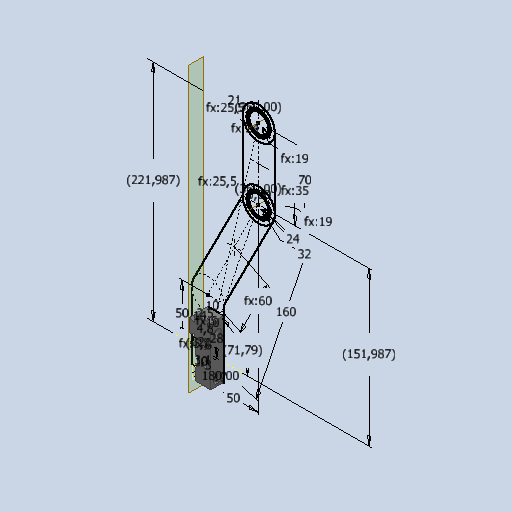
# Autodesk Inventor part: ParallelSystem_ProximalPart_Driven_Counterpart
Saved by Autodesk Inventor 2024 (Build 280153000, 153)
## iProperties
Created: 2022-07-18
Part Number: ParallelSystem_ProximalPart_Driven_Counterpart
Material: PBT-Kunststoff
Document SubType Name: Modeling
Designer: alexw
Density: 1.31 g/cm^3
Appearance: Glatt - Weiß
Mass: 124.576 g
Surface Area: 279.297 cm^2
Volume: 95.0965 cm^3
d4: 25,000 mm
d7: 5,000 mm
d9: 6,000 mm
d10: 0,00 grd
d11: 25,000 mm
d23: 8,000 mm
d36: 0,00 grd
d37: 30,000 mm
d40: 120,000 mm
d41: 50,000 mm
d42: 60,000 mm
d43: 19,000 mm
d44: 12,000 mm
d45: 35,000 mm
Passfeder_width: 3,000 mm
Nabennuttiefe: 1,400 mm
ParallelLink_BearingStep_Height: 10,000 mm
ParallelLink_Lever_Thickness: 8,000 mm
ParallelHebel_Gabelgelenk_OuterDia: 32,000 mm
Nadellager_OuterDia: 19,000 mm
ParallelHebel_Passflansch_HoleDia: 25,500 mm
d65: 3,000 oE
d69: 25,500 mm
d70: 3,000 oE
Distanze_daVinciHead_Pivot: 221,987 mm
Lager_Einbautiefe: 5,000 mm
Lager_Bohrung_Durchmesser: 19,000 mm
Support_Link_Length: 160,000 mm
ParallelMech_LINK_GabelDist: 70,000 mm
VerticalDistance: 70,000 mm
Author: alexw
Autodesk Inventor part; units mm, degrees
note: some values were not read from the file. Chosen so that the rebuilt part matches the saved one: direction of "Bohrung6".
ref_plane "YZ Plane" through (0, 0, 0) normal (1, 0, 0) x (0, 1, 0)
ref_plane "XZ Plane" through (0, 0, 0) normal (0, 1, 0) x (-1, 0, 0)
sketch "Skizze1" plane through (0, 0, 0) normal (0, 0, 1) x (1, 0, 0)
  line L0 (-33.0017, 0) -> (83.0017, 0) construction
  circle A0 centre (50, 151.9868) radius 16
  line L1 (66, 151.9868) -> (66, 221.9868)
  line L2 (34, 151.9868) -> (34, 221.9868)
  line L3 (50, 151.9868) -> (50, 237.9868) construction
  line L4 (50, 151.9868) -> (50, 167.9868) construction
  line L5 (34, 151.9868) -> (66, 151.9868) construction
  line L6 (-16, 0) -> (-16, 50)
  line L7 (16, 0) -> (16, 50)
  line L8 (-16, 50) -> (16, 50) construction
  circle A1 centre (0, 50) radius 16 construction
  line L9 (-14.2566, 57.2629) -> (34, 151.9868)
  arc A2 (-14.2566, 57.2629) -> (-16, 50) centre (0, 50) ccw
  line L10 (16, 50) -> (64.2566, 144.7239)
  arc A3 (64.2566, 144.7239) -> (66, 151.9868) centre (50, 151.9868) ccw
  line L11 (0, 50) -> (50, 151.9868) construction
  circle A4 centre (50, 221.9868) radius 16
  circle A5 centre (50, 221.9868) radius 9.5
  circle A6 centre (50, 151.9868) radius 9.5
  line L12 (0, 0) -> (0, 5) construction
  circle A7 centre (50, 151.9868) radius 12.75 construction
  circle A8 centre (50, 221.9868) radius 12.75 construction
  line L13 (0, 0) -> (50, 221.9868) construction
  circle A9 centre (50, 221.9868) radius 10.5
  circle A10 centre (50, 151.9868) radius 10.5
  circle A11 centre (50, 151.9868) radius 12
  circle A12 centre (50, 221.9868) radius 12
  line L14 (-16, 0) -> (-16, -17)
  line L15 (-16, -17) -> (16, -17)
  line L16 (16, -17) -> (16, 0)
  circle A13 centre (0, 0) radius 5
  line L17 (-1.5, -4.7697) -> (-1.5, -17)
  line L18 (1.5, -17) -> (1.5, -4.7697)
  line L19 (-16, 0) -> (16, 0) construction
  arc A14 (16, 0) -> (-16, 0) centre (0, 0) ccw
  line L20 (-1.5, 4.7697) -> (-1.5, 10.7697)
  arc A15 (1.5, 10.7697) -> (-1.5, 10.7697) centre (0, 10.7697) ccw
  line L21 (1.5, 10.7697) -> (1.5, 4.7697)
  line L22 (1.5, 4.7697) -> (-1.5, 4.7697)
  line L23 (0, 12.2697) -> (0, 40)
  line L24 (0, 40) -> (16, 40)
  line L25 (0, 33) -> (-4.8, 35)
  line L26 (-4.8, 35) -> (-4.8, 21)
  line L27 (-4.8, 21) -> (0, 23)
  line L28 (-4.8, 28) -> (0, 28) construction
  line L29 (-4.8, 30.5) -> (0, 30.5) construction
  line L30 (-4.8, 25.5) -> (0, 25.5) construction
  circle A16 centre (-10.5, 0) radius 1.55
  circle A17 centre (10.5, 0) radius 1.55
  line L31 (0, 0) -> (50, 151.9868) construction
  point P0 (26.4122, 103.8739)
  point P1 (50, 186.9868)
  point P2 (50, 164.7368)
  point P3 (38.9582, 145.6118)
  point P4 (61.0418, 145.6118)
  point P5 (50, 234.7368)
  point P6 (38.9582, 215.6118)
  point P7 (61.0418, 215.6118)
  point P8 (-5, 0)
  dimension "d69" = 25.5
  dimension "ParallelHebel_Passflansch_HoleDia" = 25.5
  dimension "d36" = 0
  dimension "ParallelHebel_Gabelgelenk_OuterDia" = 32
  dimension "VerticalDistance" = 70
  dimension "d42" = 60
  dimension "d43" = 19
  dimension "Nadellager_OuterDia" = 19
  dimension "d45" = 35
  dimension "d67" = 360
  dimension "d72" = 360
  dimension "Distanze_daVinciHead_Pivot" = 221.9868
  dimension "d88" = 21
  dimension "d91" = 24
  dimension "d92" = 24
  dimension "d97" = 151.9868
  dimension "Support_Link_Length" = 160
  dimension "d100" = 10
  dimension "d101" = 3
  dimension "d102" = 0
  dimension "d103" = 17
  dimension "d105" = 32
  dimension "d125" = 50
  dimension "d128" = 50
  dimension "d138" = 6
  dimension "d139" = 10
  dimension "d142" = 14
  dimension "d143" = 10
  dimension "d144" = 2.5
  dimension "d145" = 5
  dimension "d146" = 4.8
  dimension "d147" = 28
  dimension "d173" = 11
  dimension "d174" = 5.5
  dimension "d175" = 3.1
  dimension "d178" = 71.79
  constraints: 62 end point, 26 point on circle, 22 point on line, 16 centre point, 16 tangent, 12 coincident, 9 perpendicular, 5 vertical, 4 midpoint, 3 equal length, 3 equal radius, 3 horizontal, 3 parallel, 2 collinear, 2 symmetric about line, 2 vertical alignment, 13 other
  measures "d36" distance between parallel lines of L3 L4
  measures "ParallelHebel_Gabelgelenk_OuterDia" diameter of A0
  measures "VerticalDistance" distance of A4.centre point (50, 151.987)
  measures "d42" distance of point (26.412, 103.874) A1.centre
  measures "d43" diameter of A5
  measures "Nadellager_OuterDia" diameter of A6
  measures "d45" distance of point (50, 186.987) point (50, 151.987)
  measures "Distanze_daVinciHead_Pivot" distance from line of A4.centre L0
  measures "d88" diameter of A9
  measures "d91" diameter of A11
  measures "d92" diameter of A12
  measures "d97" vertical distance of point (50, 151.987) L12.start
  measures "Support_Link_Length" distance of A0.centre L12.start
  measures "d100" diameter of A13
  measures "d101" distance between parallel lines of L18 L17
  measures "d102" angle of L16 L14
  measures "d103" distance between parallel lines of L15 L19
  measures "d105" diameter of A14
  measures "d125" distance of L12.start L11.start
  measures "d128" horizontal distance of L12.start point (50, 151.987)
  measures "d138" distance from line of L22 A15.centre
  measures "d139" distance between parallel lines of L8 L24
  measures "d142" distance of L25.end L26.end
  measures "d143" distance of L27.end L25.start
  measures "d144" distance between parallel lines of L29 L28
  measures "d145" distance between parallel lines of L29 L30
  measures "d146" distance between parallel lines of L23 L26
  measures "d147" distance from line of L12.start L28
  measures "d173" distance of L6.start point (-5, 0)
  measures "d174" distance from line of L14 point (-10.5, 0)
  measures "d175" diameter of A16
  measures "d178" angle of L0 L31
extrude "Extrusion2" add sketch "Skizze1" along normal blind 8 contours A0 | A0 L2 A4 L1 | A0 L10 L7 L24 L23 L25 L26 L27 A14 L6 A2 L9 | A4 | L7 A14 L23 L24 | A14 L23 A15 L20 A13 L17 L15 L14 | L16 L15 L18 A13 L21 A15 L23 A14 | L23 L27 L26 L25 | A15 L21 A13 L20 | A9 | A10 | A11 | A12 | A16 | A17
fillet "Rundung1" radius 25 2 edges at (34, 151.9868, 4) (16, 50, 4)
hole "Bohrung2" at (50, 186.9868, 0) at (26.4122, 103.8739, 0) direction (0, 0, 1) diameter 8 end through all
ref_plane "Arbeitsebene1" through (50, 151.9868, 0) normal (-1, 0, 0) x (0, 0, 1)
extrude "Extrusion6" cut sketch "Skizze1" along normal blind 1 contours A5 | A9 | A10 | A11 | A12
extrude "Extrusion7" cut sketch "Skizze1" along normal blind 1 from surface at 1 contours A9 | A10
sketch "Skizze8" plane through (0, 0, 8) normal (0, 0, 1) x (1, 0, 0)
  circle A0 centre (50, 186.9868) radius 4 projected
  circle A1 centre (26.4122, 103.8739) radius 4 projected
  arc A2 (64.2566, 144.7239) -> (66, 151.9868) centre (50, 151.9868) ccw projected
  line L0 (66, 151.9868) -> (66, 221.9868) projected
  arc A3 (66, 221.9868) -> (34, 221.9868) centre (50, 221.9868) ccw projected
  line L1 (34, 221.9868) -> (34, 157.988) projected
  arc A4 (31.2759, 146.6396) -> (34, 157.988) centre (9, 157.988) ccw projected
  line L2 (31.2759, 146.6396) -> (-14.2566, 57.2629) projected
  arc A5 (-14.2566, 57.2629) -> (-16, 50) centre (0, 50) ccw projected
  line L3 (-16, 50) -> (-16, -17) projected
  line L4 (-16, -17) -> (-1.5, -17) projected
  line L5 (-1.5, -17) -> (-1.5, -4.7697) projected
  arc A6 (1.5, -4.7697) -> (-1.5, -4.7697) centre (0, 0) ccw projected
  line L6 (1.5, -4.7697) -> (1.5, -17) projected
  line L7 (1.5, -17) -> (16, -17) projected
  line L8 (16, -17) -> (16, 43.9989) projected
  arc A7 (18.7241, 55.3472) -> (16, 43.9989) centre (41, 43.9989) ccw projected
  line L9 (18.7241, 55.3472) -> (64.2566, 144.7239) projected
  circle A8 centre (50, 151.9868) radius 9.5 projected
  circle A9 centre (50, 221.9868) radius 9.5 projected
extrude "Extrusion9" add sketch "Skizze8" along normal blind 5
sketch "Skizze5" plane through (-1.5, -17, 0) normal (1, 0, 0) x (0, 0, -1)
  line L0 (0, 0) -> (0, 12.2303) construction
  line L1 (0, 12.2303) -> (-13, 12.2303) construction
  line L2 (0, 0) -> (-13, 0) construction
  line L3 (-13, 12.2303) -> (0, 0) construction
  line L4 (-13, 0) -> (0, 12.2303) construction
  line L5 (-13, 0) -> (-13, 12.2303) construction
  point P0 (0, 17)
  point P1 (-6.5, 6.1152)
  constraints: 4 end point, 1 midpoint
extrude "Extrusion11" add sketch "Skizze1" along normal up to surface (13 mm away) separate body contours L7 A14 L23 L24 | L16 L15 L18 A13 L21 A15 L23 A14 | L23 L27 L26 L25 | A17
extrude "Extrusion10" cut sketch "Skizze1" along normal up to surface (13 mm away) contours L7 A14 L23 L24 | L16 L15 L18 A13 L21 A15 L23 A14 | L23 L27 L26 L25 | A15 L21 A13 L20 | A17 bodies 1
hole "Bohrung4" at (-1.5, -10.8848, 6.5) direction (-1, 0, 0) diameter 3.242 end through all bodies 1 thread size "M4x0.7" class "6H" standard "ISO Metric profile"
sketch "Skizze9" plane through (16, -17, 0) normal (1, 0, 0) x (0, 0, -1)
  point P0 (0, 17)
  point P1 (-6.5, 6.1152)
hole "Bohrung6" at (16, -10.8848, 6.5) direction (-1, 0, 0) diameter 4.5 depth 17.5 counterbore diameter 8 counterbore depth 4.5 bodies 2 clearance for "Inbusschraube DIN EN ISO 4762" size "M4" standard "DIN"
ref_plane "Arbeitsebene2" through (-4.8, 72.7467, 13) normal (-1, 0, 0) x (0, 1, 0)
sketch "Skizze12" plane through (-4.8, 72.7467, 13) normal (-1, 0, 0) x (0, 1, 0)
  line L0 (-44.7467, 13) -> (-44.7467, 6.5) construction
  line L1 (-22.7467, 13) -> (-89.7467, 13) construction
  line L2 (-22.7467, 0) -> (-89.7467, 0) construction
  point P0 (-72.7467, 13)
  point P1 (-44.7467, 13)
  dimension "d150" = 13
  dimension "d151" = 6.5
  constraints: 2 end point, 1 coincident, 1 vertical
  measures "d150" distance between parallel lines of L1 L2
  measures "d151" distance of L0.start L0.end
sketch "Skizze13" plane through (16, -17, 0) normal (1, 0, 0) x (0, 0, -1)
  point P0 (0, 17)
  point P1 (-6.5, 45)
hole "Bohrung7" at (-4.8, 28, 6.5) direction (-1, 0, 0) diameter 3.242 end through all bodies 1 thread size "M4x0.7" class "6H" standard "ISO Metric profile"
hole "Bohrung8" at (16, 28, 6.5) direction (-1, 0, 0) diameter 4.5 end through all counterbore diameter 8 counterbore depth 4.5 bodies 2 clearance for "Inbusschraube DIN EN ISO 4762" size "M4" standard "DIN"
extrude "Extrusion12" cut sketch "Skizze1" along normal through all contours A17 bodies 2
delete faces "Fläche löschen1" heal no whole lump yes faces at (-8.5333, 28.26, 4.9)
thicken "Thicken1" operation add thickness 0.15 both sides no extend neighbours yes toward (-0.3846154, -0.9230769, 0) bodies 2 faces at (-1.6, 33.6667, 4.3333) (-4.8, 22.5888, 6.5904) (-3.2, 21.6667, 4.3333) (0, 19.4232, 8.6667) (0, 37.6667, 4.3333)
equation "\"NKX_10_RiadialPart_Dia\" = 19"
equation "\"Lager_Bohrung_Durchmesser\" = 19"
equation "\"Lager_Einbautiefe\" = 5"
